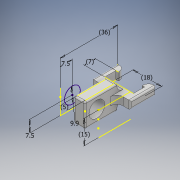
# Autodesk Inventor part: 보조바퀴 축
Saved by Autodesk Inventor 2018 (Build 220112000, 112)
## iProperties
Created: 2019-11-18
Part Number: 보조바퀴 축
Material: 일반
Document SubType Name: Modeling
Designer: LeeYounSeo
Density: 1 g/cm^3
Appearance: 기본값
Author: LeeYounSeo
Autodesk Inventor part; units mm, degrees
ref_plane "YZ Plane" through (0, 0, 0) normal (1, 0, 0) x (0, 1, 0)
ref_plane "XZ Plane" through (0, 0, 0) normal (0, 1, 0) x (-1, 0, 0)
ref_plane "XY Plane" through (0, 0, 0) normal (0, 0, 1) x (1, 0, 0)
sketch "스케치1" plane through (0, 0, 0) normal (0, 1, 0) x (-1, 0, 0)
  point P0 (0, 0)
sketch "스케치2" plane through (0, 0, 0) normal (0, 1, 0) x (-1, 0, 0)
  line L0 (0, 0) -> (24, 0)
  line L1 (24, 0) -> (24, -5)
  line L2 (24, -5) -> (0, -5)
  line L3 (0, -5) -> (0, 0)
  dimension "d0" = 24
  dimension "d1" = 5
  constraints: 8 end point, 2 parallel, 1 horizontal, 1 perpendicular
  measures "d0" distance of L1.end L2.end
  measures "d1" distance of L0.end L1.end
extrude "돌출1" add sketch "스케치2" along normal blind 25
sketch "스케치3" plane through (0, 25, 0) normal (0, 1, 0) x (1, 0, 0)
  line L0 (-21, 0) -> (-3, 0)
  line L1 (-3, 0) -> (-3, 5)
  line L2 (-3, 5) -> (-21, 5)
  line L3 (-21, 5) -> (-21, 0)
  line L4 (0, 5) -> (-24, 5) projected
  line L5 (-24, 0) -> (0, 0) projected
  line L6 (-24, 5) -> (-24, 0) projected
  line L7 (0, 0) -> (0, 5) projected
  dimension "d4" = 3
  dimension "d5" = 3
  constraints: 8 end point, 2 collinear, 2 parallel, 1 horizontal, 1 perpendicular
  measures "d4" distance between parallel lines of L3 L6
  measures "d5" distance between parallel lines of L7 L1
extrude "돌출2" add sketch "스케치3" along normal blind 11 contours L5 L6 L4 L3 | L1 L4 L7 L5
sketch "스케치4" plane through (-21, 25, 0) normal (1, 0, 0) x (0, 0, -1)
  line L0 (0, 0) -> (0, 11) projected
  line L1 (5, 11) -> (0, 11)
  line L2 (0, 11) -> (0, 7)
  line L3 (0, 7) -> (5, 7)
  line L4 (5, 7) -> (5, 11)
  point P0 (0, -25)
  dimension "d8" = 4
  constraints: 8 end point, 2 parallel, 1 horizontal, 1 perpendicular, 1 point on line
  measures "d8" distance of L1.end L2.end
extrude "돌출3" add sketch "스케치4" along normal blind 1.5
sketch "스케치5" plane through (-3, 25, -5) normal (-1, 0, 0) x (0, 0, 1)
  line L0 (0, 11) -> (5, 11) projected
  line L1 (5, 11) -> (0, 11)
  line L2 (0, 11) -> (0, 7)
  line L3 (0, 7) -> (5, 7)
  line L4 (5, 7) -> (5, 11)
  point P0 (5, -25)
  dimension "d11" = 4
  constraints: 8 end point, 2 parallel, 1 horizontal, 1 perpendicular
  measures "d11" distance of L1.end L2.end
extrude "돌출4" add sketch "스케치5" along normal blind 1.5
sketch "스케치6" plane through (-24, 0, 0) normal (0, 0, 1) x (1, 0, 0)
  line L0 (0, 0) -> (24, 0) projected
  line L1 (0, 0) -> (0, 36) projected
  line L2 (24, 0) -> (0, 0)
  line L3 (0, 0) -> (0, 20)
  line L4 (0, 20) -> (24, 20)
  line L5 (24, 20) -> (24, 0)
  line L6 (3, 25) -> (21, 25) projected
  dimension "d14" = 5
  constraints: 8 end point, 2 parallel, 1 horizontal, 1 perpendicular, 1 point on line
  measures "d14" distance between parallel lines of L4 L6
extrude "돌출5" add sketch "스케치6" along normal blind 5
sketch "스케치7" plane through (0, 0, -5) normal (0, 0, -1) x (-1, 0, 0)
  line L0 (0, 20) -> (24, 20)
  line L1 (24, 20) -> (24, 0)
  line L2 (24, 0) -> (0, 0)
  line L3 (0, 0) -> (0, 20)
  line L4 (0, 0) -> (0, 36) projected
  line L5 (24, 0) -> (24, 36) projected
  line L6 (24, 0) -> (0, 0) projected
  line L7 (3, 25) -> (21, 25) projected
  dimension "d17" = 5
  constraints: 8 end point, 3 collinear, 2 parallel, 1 horizontal, 1 perpendicular
  measures "d17" distance between parallel lines of L0 L7
extrude "돌출6" add sketch "스케치7" along normal blind 5
sketch "스케치8" plane through (0, 36, 0) normal (1, 0, 0) x (0, 0, -1)
  line L0 (10, -16) -> (10, -36) projected
  line L1 (-5, -36) -> (-5, -16) projected
  point P0 (0, -36)
  dimension "d20" = 15
  measures "d20" distance between parallel lines of L0 L1
sketch "스케치9" plane through (-24, 36, -5) normal (-1, 0, 0) x (0, 0, 1)
  circle A0 centre (2.5, -28.5) radius 4.95
  line L0 (-5, -36) -> (-5, -16) projected
  line L1 (10, -36) -> (-5, -36) projected
  line L2 (0, 0) -> (5, 0) projected
  point P0 (5, -36)
  dimension "d21" = 9.9
  dimension "d22" = 7.5
  dimension "d23" = 7.5
  dimension "d24" = 36
  constraints: 1 centre point
  measures "d21" diameter of A0
  measures "d22" distance from line of L0 A0.centre
  measures "d23" distance from line of L1 A0.centre
  measures "d24" distance between parallel lines of L2 L1
sketch "스케치10" plane through (-24, 36, -5) normal (-1, 0, 0) x (0, 0, 1)
  line L0 (0, -16) -> (-5, -16) projected
  line L1 (-5, -36) -> (10, -36) projected
  line L2 (-5, -16) -> (10, -16)
  line L3 (10, -16) -> (10, -36)
  line L4 (10, -36) -> (-5, -36)
  line L5 (-5, -36) -> (-5, -16)
  circle A0 centre (2.5, -28.5) radius 4.95 projected
  point P0 (5, -36)
  constraints: 8 end point, 2 parallel, 1 horizontal, 1 perpendicular
extrude "돌출7" cut sketch "스케치10" against normal blind 50 contours A0
sketch "스케치11" plane through (-24, 36, -5) normal (-1, 0, 0) x (0, 0, 1)
  line L0 (0, -16) -> (-5, -16) projected
  line L1 (10, -16) -> (10, -36) projected
  line L2 (-5, -16) -> (10, -16)
  line L3 (10, -16) -> (10, -36)
  line L4 (10, -36) -> (-5, -36)
  line L5 (-5, -36) -> (-5, -16)
  point P0 (5, -36)
  constraints: 8 end point, 2 parallel, 1 horizontal, 1 perpendicular
extrude "돌출8" cut sketch "스케치11" against normal blind 8.5
sketch "스케치12" plane through (0, 36, 0) normal (1, 0, 0) x (0, 0, -1)
  line L0 (0, -16) -> (-5, -16) projected
  line L1 (10, -36) -> (10, -16) projected
  line L2 (-5, -16) -> (10, -16)
  line L3 (10, -16) -> (10, -36)
  line L4 (10, -36) -> (-5, -36)
  line L5 (-5, -36) -> (-5, -16)
  point P0 (0, -36)
  constraints: 8 end point, 2 parallel, 1 horizontal, 1 perpendicular
extrude "돌출9" cut sketch "스케치12" against normal blind 8.5
sketch "스케치13" plane through (-24, 0, 5) normal (0, 0, 1) x (1, 0, 0)
  point P0 (24, 0)
fillet "모깎기1" radius 4 4 edges at (-12, 20, 0) (-15.5, 20, -2.5) (-12, 20, -5) (-8.5, 20, -2.5)
fillet "모깎기2" radius 1 18 edges at (-8.5, 10, -10) (-8.5, 10, 5) (-8.5, 0, -2.5) (-15.5, 10, -10) (-12, 20, -10) (-12, 20, 5) (-15.5, 10, 5) (-15.5, 0, -2.5) (-12, 0, 5) (-12, 0, -10) (0, 20, -2.5) (0, 36, -2.5) (0, 28, -5) (0, 28, 0) (-24, 28, 0) (-24, 28, -5) (-24, 20, -2.5) (-24, 36, -2.5)
fillet "모깎기3" radius 3.5 2 edges at (-4.5, 36, -2.5) (-19.5, 36, -2.5)
sketch "스케치14" plane through (-3, 25, -5) normal (0, 0, -1) x (-1, 0, 0)
  line L0 (18, 7) -> (18, 0) projected
  line L1 (0, 0) -> (0, 7) projected
  point P0 (-3, -25)
  dimension "d34" = 18
  measures "d34" distance between parallel lines of L0 L1
sketch "스케치15" plane through (-21, 25, 0) normal (0, 0, 1) x (1, 0, 0)
  line L0 (0, 7) -> (1.5, 7) projected
  line L1 (0, 0) -> (18, 0) projected
  point P0 (21, -25)
  dimension "d35" = 7
  measures "d35" distance between parallel lines of L0 L1
sketch "스케치16" plane through (-24, 0, 5) normal (0, 0, 1) x (1, 0, 0)
  line L0 (14.5, 19) -> (14.5, 1) projected
  line L1 (9.5, 1) -> (9.5, 19) projected
  point P0 (24, 0)
  dimension "d36" = 5
  measures "d36" distance between parallel lines of L0 L1
sketch "스케치17" plane through (-8.5, 36, 0) normal (1, 0, 0) x (0, 0, -1)
  point P0 (0, -36)
